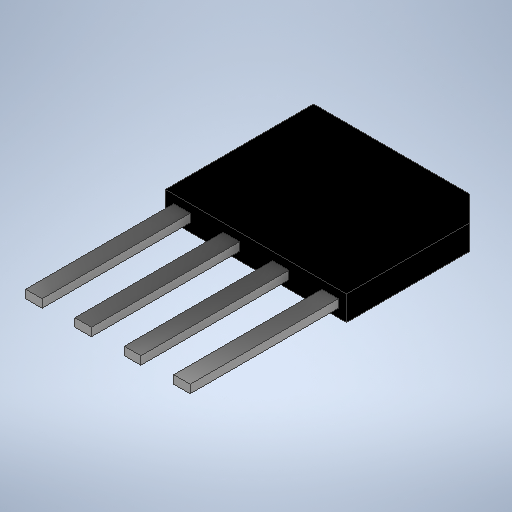
# Autodesk Inventor part: Rectifier
Saved by Autodesk Inventor 2025.2 (Build 292293000, 293)
## iProperties
Created: 2025-04-04
Part Number: Rectifier
Material: Generic
Document SubType Name: Modeling
Designer: joaki
Density: 1 g/cm^3
Appearance: Default
Author: joaki
Autodesk Inventor part; units mm, degrees
ref_plane "YZ Plane" through (0, 0, 0) normal (1, 0, 0) x (0, 1, 0)
ref_plane "XZ Plane" through (0, 0, 0) normal (0, 1, 0) x (-1, 0, 0)
ref_plane "XY Plane" through (0, 0, 0) normal (0, 0, 1) x (1, 0, 0)
sketch "Sketch1" plane through (0, 0, 0) normal (0, 1, 0) x (-1, 0, 0)
  line L0 (9.8262, 5.9604) -> (-12.1738, 5.9604)
  line L1 (-12.1738, 5.9604) -> (-12.1738, -12.0396)
  line L2 (-12.1738, -12.0396) -> (9.8262, -12.0396)
  line L3 (9.8262, -12.0396) -> (9.8262, 5.9604)
  point P0 (0, 0)
  dimension "d0" = 22
  dimension "d1" = 18
  constraints: 8 end point, 2 parallel, 1 horizontal, 1 perpendicular
  measures "d0" distance of L1.end L2.end
  measures "d1" distance of L2.end L0.start
extrude "Extrusion1" add sketch "Sketch1" along normal blind 3
sketch "Sketch2" plane through (-9.8262, 0, 5.9604) normal (0, 0, 1) x (1, 0, 0)
  line L0 (1, 2) -> (3, 2)
  line L1 (3, 2) -> (3, 1)
  line L2 (3, 1) -> (1, 1)
  line L3 (1, 1) -> (1, 2)
  line L4 (0, 3) -> (22, 3) projected
  line L5 (0, 0) -> (0, 3) projected
  line L6 (7, 2) -> (9, 2)
  line L7 (9, 2) -> (9, 1)
  line L8 (9, 1) -> (7, 1)
  line L9 (7, 1) -> (7, 2)
  line L10 (13, 2) -> (15, 2)
  line L11 (15, 2) -> (15, 1)
  line L12 (15, 1) -> (13, 1)
  line L13 (13, 1) -> (13, 2)
  line L14 (19, 2) -> (21, 2)
  line L15 (21, 2) -> (21, 1)
  line L16 (21, 1) -> (19, 1)
  line L17 (19, 1) -> (19, 2)
  line L18 (22, 0) -> (22, 3) projected
  point P0 (9.8262, 0)
  point P1 (1, 1.5)
  point P2 (7, 1.5)
  point P3 (13, 1.5)
  point P4 (19, 1.5)
  point P5 (8, 2)
  dimension "d4" = 1
  dimension "d5" = 1
  dimension "d6" = 2
  dimension "d7" = 1
  dimension "d8" = 1
  dimension "d9" = 2
  dimension "d10" = 1
  dimension "d11" = 2
  dimension "d12" = 1
  dimension "d13" = 2
  dimension "d14" = 1
  dimension "d15" = 1
  dimension "d16" = 1
  dimension "d17" = 1
  dimension "d18" = 4
  dimension "d19" = 4
  constraints: 32 end point, 8 parallel, 5 midpoint, 4 horizontal, 4 perpendicular
  measures "d4" distance between parallel lines of L0 L2
  measures "d5" distance between parallel lines of L4 L0
  measures "d6" distance of L0.start L0.end
  measures "d7" distance from line of L5 point (1, 1.5)
  measures "d8" distance between parallel lines of L6 L8
  measures "d9" distance of L6.start L6.end
  measures "d10" distance between parallel lines of L10 L12
  measures "d11" distance of L10.start L10.end
  measures "d12" distance between parallel lines of L14 L16
  measures "d13" distance of L14.start L14.end
  measures "d14" distance from line of L4 point (8, 2)
  measures "d15" distance between parallel lines of L4 L10
  measures "d16" distance between parallel lines of L4 L14
  measures "d17" distance between parallel lines of L18 L15
  measures "d18" distance between parallel lines of L17 L11
  measures "d19" distance between parallel lines of L9 L1
extrude "Extrusion2" add sketch "Sketch2" along normal blind 18
sketch "Sketch3" plane through (0, 3, 0) normal (0, 1, 0) x (1, 0, 0)
  line L0 (12.1738, 12.0396) -> (9.1738, 12.0396)
  line L1 (12.1738, 12.0396) -> (-9.8262, 12.0396) projected
  line L2 (12.1738, 12.0396) -> (12.1738, 9.0396)
  line L3 (12.1738, 9.0396) -> (9.1738, 12.0396)
  point P0 (0, 0)
  dimension "d22" = 3
  dimension "d23" = 3
  constraints: 6 end point, 1 perpendicular, 1 point on line
  measures "d22" distance of L0.start L0.end
  measures "d23" distance of L0.start L2.end
extrude "Extrusion3" cut sketch "Sketch3" against normal blind 18
body "Solid1"
